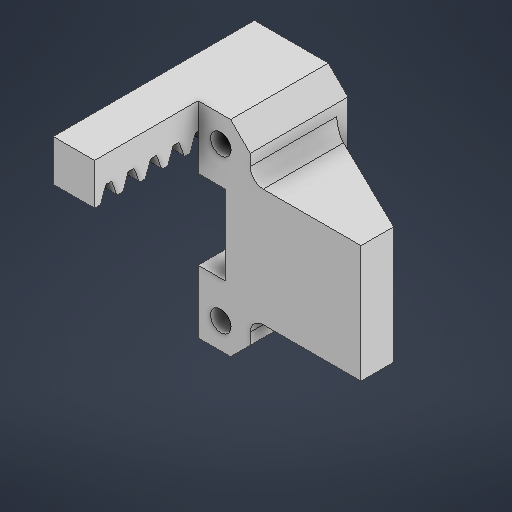
# Autodesk Inventor part: GA_1
Saved by Autodesk Inventor 2025.2 (Build 292293000, 293)
## iProperties
Created: 2025-06-17
Part Number: GA_1
Material: Generic
Document SubType Name: Modeling
Designer: Tiago
Density: 1 g/cm^3
Appearance: Default
Author: Tiago
Autodesk Inventor part; units mm, degrees
ref_plane "YZ Plane" through (0, 0, 0) normal (1, 0, 0) x (0, 1, 0)
ref_plane "XZ Plane" through (0, 0, 0) normal (0, 1, 0) x (-1, 0, 0)
sketch "Sketch1" plane through (0, 0, 0) normal (0, 0, 1) x (1, 0, 0)
  line L0 (-7.5, -9) -> (7.5, -9)
  line L1 (7.5, -9) -> (7.5, 9)
  line L2 (7.5, 9) -> (-7.5, 9)
  line L3 (-9.5, -11) -> (-9.5, -12.75)
  line L4 (-12.5, -15.75) -> (-17.5, -15.75)
  arc A0 (-7.5, -9) -> (-9.5, -11) centre (-7.5, -11) ccw
  line L5 (-12.5, -15.75) -> (-9.5, -12.75)
  line L6 (-17.5, -15.75) -> (-17.5, -6.1)
  line L7 (-17.5, -6.1) -> (-13.3, -6.1)
  line L8 (-13.3, -6.1) -> (-13.3, 0)
  line L9 (2.7531, 0) -> (-2.7531, 0) construction
  line L10 (-9.5, 11) -> (-9.5, 12.75)
  line L11 (-12.5, 15.75) -> (-17.5, 15.75)
  arc A1 (-9.5, 11) -> (-7.5, 9) centre (-7.5, 11) ccw
  line L12 (-12.5, 15.75) -> (-9.5, 12.75)
  line L13 (-17.5, 15.75) -> (-17.5, 6.1)
  line L14 (-17.5, 6.1) -> (-13.3, 6.1)
  line L15 (-13.3, 6.1) -> (-13.3, 0)
  circle A2 centre (-14, -11.75) radius 1.575
  circle A3 centre (-14, 11.75) radius 1.575
  line L16 (-17.5, 15.75) -> (-23.85, 15.75)
  line L17 (-23.85, 15.75) -> (-23.85, 9.4)
  line L18 (-23.85, 9.4) -> (-17.5, 9.4)
  line L19 (-9.5, 11.875) -> (-9.5, -11.875)
  point P0 (0, 0)
  point P1 (0, 0)
  point P2 (7.5, 0)
  point P3 (0, -9)
  point P4 (-9.5, -15.75)
  point P5 (0, 0)
  point P6 (-9.5, 15.75)
  dimension "d1" = 18
  dimension "d3" = 8
  dimension "d4" = 2
  dimension "d5" = 3
  dimension "d6" = 3
  dimension "d7" = 9.65
  dimension "d8" = 4.2
  dimension "d9" = 6.1
  dimension "d10" = 7.5
  dimension "d11" = 3.875
  dimension "d12" = 3.15
  dimension "d13" = 3.5
  dimension "d14" = 4
  dimension "d15" = 6.35
  dimension "d16" = 6.35
  constraints: 40 end point, 11 symmetric about line, 5 horizontal, 5 point on line, 5 vertical, 4 centre point, 4 coincident, 4 midpoint, 4 point on circle, 2 perpendicular, 2 tangent, 1 horizontal alignment, 1 parallel, 1 vertical alignment, 2 other
  measures "d1" distance of L0.end L1.end
  measures "d3" distance of point (-9.5, -15.75) L4.end
  measures "d4" radius of A0
  measures "d5" distance of L4.start point (-9.5, -15.75)
  measures "d6" distance of L3.end point (-9.5, -15.75)
  measures "d7" distance of L4.end L6.end
  measures "d8" distance of L6.end L7.end
  measures "d9" distance of L7.end L8.end
  measures "d10" distance of point (0, 0) point (7.5, 0)
  measures "d11" distance of L19.end point (-9.5, -15.75)
  measures "d12" diameter of A2
  measures "d13" distance from line of L6 A2.centre
  measures "d14" distance from line of L4 A2.centre
  measures "d15" distance of L13.start L16.end
  measures "d16" distance of L16.end L17.end
extrude "Extrusion1" add sketch "Sketch1" against normal blind 15 contours L3 L5 L4 L6 L7 L8 L15 L14 L13 L11 L12 L10 L19
extrude "Extrusion2" add sketch "Sketch1" against normal blind 13.291 contours A0 L19 A1 L2 L1 L0
chamfer "Chamfer1" distance 17 distance2 8.281 1 edges at (7.5, 0, -13.291) measured on face at (-2.5, 3, -13.291)
extrude "Extrusion3" add sketch "Sketch1" along normal blind 15.861 and the other way blind 15 contours L13 L18 L17 L16
ref_plane "Work Plane1" through (-17.5, 9.4, 0) normal (1, 0, 0) x (0, 0, -1)
sketch "Sketch2" plane through (-17.5, 9.4, 0) normal (1, 0, 0) x (0, 0, -1)
  line L0 (0, 6.35) -> (0, 0) projected
  line L1 (15, 0) -> (0, 0) projected
  line L2 (15, 6.35) -> (15, 0) projected
  line L3 (0, 6.35) -> (15, 6.35) projected
  line L4 (-15.861, 6.35) -> (0, 6.35) projected
  line L5 (-15.861, 0) -> (-15.861, 6.35) projected
  line L6 (0, 0) -> (-15.861, 0) projected
  line L7 (0, -3.3) -> (0, 0) projected
  line L8 (15, -3.3) -> (0, -3.3) projected
  line L9 (15, 0) -> (15, -3.3) projected
  line L10 (0, -15.5) -> (15, -15.5) projected
  line L11 (15, -15.5) -> (15, -25.15) projected
  line L12 (15, -25.15) -> (0, -25.15) projected
  line L13 (0, -25.15) -> (0, -15.5) projected
  line L14 (-15.861, 0) -> (-14.969, 0)
  line L15 (-14.969, 0) -> (-14.1416, 2.2732)
  line L16 (-14.1416, 2.2732) -> (-13.2496, 2.2732)
  line L17 (-13.2496, 2.2732) -> (-12.4223, 0)
  line L18 (-15.861, 0) -> (15, 0) projected
  line L19 (-9.8106, 2.2732) -> (-8.9833, 0)
  line L20 (-10.7026, 2.2732) -> (-9.8106, 2.2732)
  line L21 (-11.53, 0) -> (-10.7026, 2.2732)
  line L22 (-12.422, 0) -> (-11.53, 0)
  line L23 (-6.3716, 2.2732) -> (-5.5443, 0)
  line L24 (-7.2636, 2.2732) -> (-6.3716, 2.2732)
  line L25 (-8.091, 0) -> (-7.2636, 2.2732)
  line L26 (-8.983, 0) -> (-8.091, 0)
  line L27 (-2.9326, 2.2732) -> (-2.1053, 0)
  line L28 (-3.8246, 2.2732) -> (-2.9326, 2.2732)
  line L29 (-4.652, 0) -> (-3.8246, 2.2732)
  line L30 (-5.544, 0) -> (-4.652, 0)
  line L31 (0.5064, 2.2732) -> (1.3337, 0)
  line L32 (-0.3856, 2.2732) -> (0.5064, 2.2732)
  line L33 (-1.213, 0) -> (-0.3856, 2.2732)
  line L34 (-2.105, 0) -> (-1.213, 0)
  line L35 (3.9454, 2.2732) -> (4.7727, 0)
  line L36 (3.0534, 2.2732) -> (3.9454, 2.2732)
  line L37 (2.226, 0) -> (3.0534, 2.2732)
  line L38 (1.334, 0) -> (2.226, 0)
  line L39 (7.3844, 2.2732) -> (8.2117, 0)
  line L40 (6.4924, 2.2732) -> (7.3844, 2.2732)
  line L41 (5.665, 0) -> (6.4924, 2.2732)
  line L42 (4.773, 0) -> (5.665, 0)
  line L43 (10.8234, 2.2732) -> (11.6507, 0)
  line L44 (9.9314, 2.2732) -> (10.8234, 2.2732)
  line L45 (9.104, 0) -> (9.9314, 2.2732)
  line L46 (8.212, 0) -> (9.104, 0)
  line L47 (14.2624, 2.2732) -> (15.0897, 0)
  line L48 (13.3704, 2.2732) -> (14.2624, 2.2732)
  line L49 (12.543, 0) -> (13.3704, 2.2732)
  line L50 (11.651, 0) -> (12.543, 0)
  point P0 (0, -9.4)
  point P1 (15, 0.2465)
  point P2 (11.6507, 0)
  point P3 (8.2117, 0)
  point P4 (4.7727, 0)
  point P5 (1.3337, 0)
  point P6 (-2.1053, 0)
  point P7 (-5.5443, 0)
  point P8 (-8.9833, 0)
  point P9 (-12.4223, 0)
  dimension "d29" = 0.892
  dimension "d30" = 110
  dimension "d31" = 110
  dimension "d32" = 0.892
  dimension "d33" = 2.2732
  dimension "d36" = 3.439
  constraints: 72 end point, 2 point on line, 1 horizontal, 1 parallel, 72 other
  measures "d29" distance of L5.start L14.end
  measures "d30" angle of L16 L15
  measures "d31" angle of L16 L17
  measures "d32" distance of L15.end L16.end
  measures "d33" distance between parallel lines of L6 L16
  measures "d36" distance of L17.end L19.end
extrude "Extrusion4" cut sketch "Sketch2" against normal up to surface (6.35 mm away) contours L32 L31 L1 L0 | L0 L6 L33 L32 | L2 L1 L49 L48 L47 | L15 L16 L17 L6 | L37 L36 L35 L1 | L6 L29 L28 L27 | L1 L45 L44 L43 | L21 L20 L19 L6 | L41 L40 L39 L1 | L6 L25 L24 L23
fillet "Fillet1" radius 0.2 35 edges at (-20.675, 11.6732, 14.1416) (-20.675, 11.6732, 13.2496) (-20.675, 9.4, 14.969) (-20.675, 9.4, 12.4223) (-20.675, 9.4, 11.53) (-20.675, 11.6732, 10.7026) (-20.675, 11.6732, 9.8106) (-20.675, 9.4, 8.9833) (-20.675, 9.4, 8.091) (-20.675, 11.6732, 7.2636) (-20.675, 11.6732, 6.3716) (-20.675, 9.4, 5.5443) (-20.675, 9.4, 4.652) (-20.675, 11.6732, 3.8246) (-20.675, 11.6732, 2.9326) (-20.675, 9.4, 2.1053) (-20.675, 9.4, 1.213) (-20.675, 11.6732, 0.3856) (-20.675, 11.6732, -0.5064) (-20.675, 9.4, -1.3337) (-20.675, 9.4, -2.226) (-20.675, 11.6732, -3.0534) (-20.675, 11.6732, -3.9454) (-20.675, 9.4, -4.7727) (-20.675, 9.4, -5.665) (-20.675, 11.6732, -6.4924) (-20.675, 11.6732, -7.3844) (-20.675, 9.4, -8.2117) (-20.675, 9.4, -9.104) (-20.675, 11.6732, -9.9314) (-20.675, 11.6732, -10.8234) (-20.675, 9.4, -11.6507) (-20.675, 9.4, -12.543) (-20.675, 11.6732, -13.3704) (-20.675, 11.6732, -14.2624)
equation "\"d6\" = d5"
body "Solid1"
